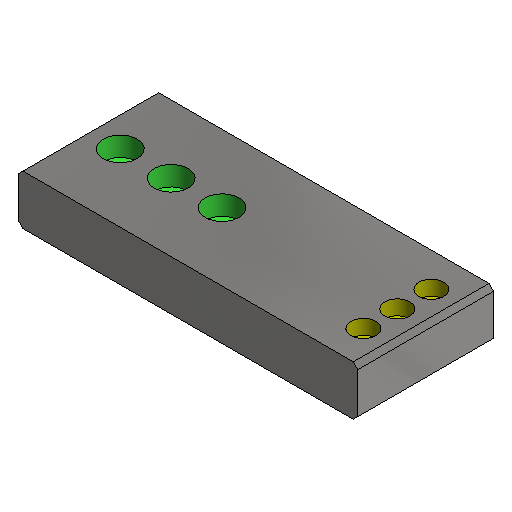
# Autodesk Inventor part: TL20240901-10320CV-021
Saved by Autodesk Inventor 2022.5 (Build 265521000, 521)
## iProperties
Category: FOLLOWER UNIT ASSY
Company: 현대 트랜시스
RuleStatus: InUse
Part Number: TL20240901-10320CV-021
Project: MEa-PJT 2LINE
Checked By: 김형민
Engr Approved By: 김형민
User Status: 2 x6
Material: SS400
Description: 0
Document SubType Name: Modeling
Mfg Approved By: 호상태
Designer: USER106
Stock Number: 021
Density: 7.85 g/cm^3
Appearance: Plating Zinc White
Detail Description: Processed products
Title: SUPPORTER PLATE
Subject: MEa차종 시트조립2라인
Author: USER106
Revision Number: A
Autodesk Inventor part; units mm, degrees
ref_plane "YZ Plane" through (0, 0, 0) normal (1, 0, 0) x (0, 1, 0)
ref_plane "XZ Plane" through (0, 0, 0) normal (0, 1, 0) x (-1, 0, 0)
ref_plane "XY Plane" through (0, 0, 0) normal (0, 0, 1) x (1, 0, 0)
sketch "Sketch2" plane through (0, 0, 0) normal (0, 0, 1) x (1, 0, 0)
  line L0 (75, -30) -> (-75, -30)
  line L1 (-75, -30) -> (-75, 30)
  line L2 (-75, 30) -> (75, 30)
  line L3 (75, 30) -> (75, -30)
  line L4 (75, -30) -> (-75, 30) construction
  line L5 (-75, -30) -> (75, 30) construction
  point P0 (0, 0)
  dimension "d1" = 150
  dimension "d2" = 60
  constraints: 12 end point, 2 midpoint, 2 parallel, 1 horizontal, 1 perpendicular
  measures "d1" distance of L1.end L2.end
  measures "d2" distance of L0.end L1.end
extrude "Extrusion1" add sketch "Sketch2" along normal mid plane 22
sketch "Sketch3" plane through (0, 0, 11) normal (0, 0, 1) x (1, 0, 0)
  line L0 (75, -30) -> (75, 30) projected
  point P0 (0, 0)
  point P1 (62.5, 0)
  point P2 (62.5, 15)
  point P3 (62.5, -15)
  point P4 (75, 0)
  dimension "d5" = 12.5
  dimension "d6" = 30
  dimension "d7" = 15
  constraints: 2 vertical alignment, 1 horizontal alignment, 1 midpoint
  measures "d5" distance from line of L0 point (62.5, 0)
  measures "d6" distance of point (62.5, 15) point (62.5, -15)
  measures "d7" distance of point (62.5, 15) point (62.5, 0)
hole "Hole1" at (62.5, 0, 11) at (62.5, 15, 11) at (62.5, -15, 11) direction (0, 0, -1) diameter 6.6 end through all counterbore diameter 11 counterbore depth 6.5 clearance for "Socket Head Cap Screw" size "M6" standard "TS Profile"
sketch "Sketch4" plane through (0, 0, 11) normal (0, 0, 1) x (1, 0, 0)
  line L0 (-75, 30) -> (-75, -30) projected
  point P0 (0, 0)
  point P1 (-60, 0)
  point P2 (-37.5, 0)
  point P3 (-15, 0)
  point P4 (-75, 0)
  point P5 (-75, 0)
  dimension "d15" = 15
  dimension "d16" = 22.5
  dimension "d17" = 22.5
  constraints: 3 horizontal alignment, 2 midpoint
  measures "d15" distance from line of point (-60, 0) L0
  measures "d16" distance of point (-37.5, 0) point (-60, 0)
  measures "d17" distance of point (-15, 0) point (-37.5, 0)
hole "Hole2" at (-60, 0, 11) at (-37.5, 0, 11) at (-15, 0, 11) direction (0, 0, -1) diameter 9 end through all counterbore diameter 15 counterbore depth 8.6 clearance for "Socket Head Cap Screw" size "M8" standard "TS Profile"
chamfer "Chamfer2" distance 2 angle 45 4 edges at (75, 0, 11) (75, 0, -11) (-75, 0, 11) (-75, 0, -11)
equation "\"d7\" = 0.5 * d6"
equation "\"d17\" = d16"
body "Solid1"
